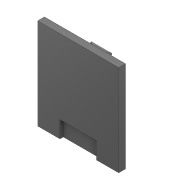
# Autodesk Inventor part: DeckelMess_Better
Saved by Autodesk Inventor 2020 (Build 240168000, 168)
## iProperties
Created: 2022-02-26
Part Number: DeckelMess_Better
Material: Acetalharz, Schwarz
Document SubType Name: Modeling
Designer: Julian Uhl
Density: 1.425 g/cm^3
Appearance: Glatt - Schwarz
Author: Julian Uhl
Autodesk Inventor part; units mm, degrees
ref_plane "YZ Plane" through (0, 0, 0) normal (1, 0, 0) x (0, 1, 0)
ref_plane "XZ Plane" through (0, 0, 0) normal (0, 1, 0) x (-1, 0, 0)
ref_plane "XY Plane" through (0, 0, 0) normal (0, 0, 1) x (1, 0, 0)
sketch "Skizze1" plane through (0, 0, 0) normal (0, 0, 1) x (1, 0, 0)
  line L0 (-24, 0) -> (144, 0) projected
  line L1 (0, -27) -> (0, 162) projected
  line L2 (0, 0) -> (120, 0)
  line L3 (120, 0) -> (120, 135)
  line L4 (120, 135) -> (0, 135)
  line L5 (0, 135) -> (0, 0)
  point P0 (0, 135)
  dimension "d0" = 135
  dimension "d1" = 120
  constraints: 8 end point, 2 parallel, 1 horizontal, 1 perpendicular
  measures "d0" distance between parallel lines of L0 L4
  measures "d1" distance between parallel lines of L3 L5
extrude "Extrusion1" add sketch "Skizze1" along normal blind 10
sketch "Skizze2" plane through (0, 0, 10) normal (0, 0, 1) x (1, 0, 0)
  line L0 (0, 0) -> (120, 0) projected
  line L1 (33, 0) -> (87, 0)
  line L2 (87, 0) -> (87, 25)
  line L3 (87, 25) -> (33, 25)
  line L4 (33, 25) -> (33, 0)
  line L5 (0, 135) -> (0, 0) projected
  dimension "d4" = 54
  dimension "d5" = 25
  dimension "d6" = 33
  constraints: 8 end point, 2 parallel, 1 horizontal, 1 perpendicular, 1 point on line
  measures "d4" distance between parallel lines of L2 L4
  measures "d5" distance between parallel lines of L0 L3
  measures "d6" distance between parallel lines of L5 L4
extrude "Extrusion2" cut sketch "Skizze2" against normal blind 5
sketch "Skizze3" plane through (0, 0, 0) normal (0, 0, -1) x (-1, 0, 0)
  line L0 (-75, 115) -> (-70, 115)
  line L1 (-70, 115) -> (-70, 110)
  line L2 (-70, 110) -> (-75, 110)
  line L3 (-75, 110) -> (-75, 115)
  line L4 (-50, 115) -> (-45, 115)
  line L5 (-45, 115) -> (-45, 110)
  line L6 (-45, 110) -> (-50, 110)
  line L7 (-50, 110) -> (-50, 115)
  line L8 (-120, 135) -> (0, 135)
  line L9 (-120, 0) -> (-120, 135) projected
  line L10 (0, 135) -> (0, 0) projected
  line L11 (-120, 135) -> (0, 135) projected
  dimension "d9" = 5
  dimension "d10" = 5
  dimension "d11" = 5
  dimension "d12" = 5
  dimension "d13" = 20
  dimension "d14" = 20
  dimension "d15" = 45
  dimension "d16" = 45
  dimension "d17" = 20
  constraints: 18 end point, 4 parallel, 2 horizontal, 2 perpendicular
  measures "d9" distance between parallel lines of L6 L4
  measures "d10" distance between parallel lines of L5 L7
  measures "d11" distance from line of L2 L0.start
  measures "d12" distance between parallel lines of L3 L1
  measures "d13" distance between parallel lines of L8 L0
  measures "d14" distance between parallel lines of L8 L4
  measures "d15" distance between parallel lines of L9 L3
  measures "d16" distance between parallel lines of L10 L5
  measures "d17" distance between parallel lines of L11 L0
extrude "Extrusion3" add sketch "Skizze3" along normal blind 20
sketch "Skizze4" plane through (75, 110, 0) normal (1, 0, 0) x (0, 0, -1)
  line L0 (0, 5) -> (20, 5) projected
  line L1 (20, 5) -> (25, 5)
  line L2 (25, 5) -> (25, 0)
  line L3 (25, 0) -> (20, 0)
  line L4 (20, 0) -> (20, 5)
  point P0 (0, -110)
  dimension "d20" = 5
  dimension "d21" = 5
  constraints: 8 end point, 2 parallel, 1 horizontal, 1 perpendicular
  measures "d20" distance between parallel lines of L2 L4
  measures "d21" distance between parallel lines of L1 L3
extrude "Extrusion4" add sketch "Skizze4" against normal blind 30
fillet "Rundung1" radius 2.5 12 edges at (60, 110, -25) (60, 115, -25) (75, 115, -12.5) (75, 110, -12.5) (45, 110, -12.5) (50, 110, -10) (70, 110, -10) (60, 110, -20) (50, 115, -10) (60, 115, -20) (70, 115, -10) (45, 115, -12.5)
